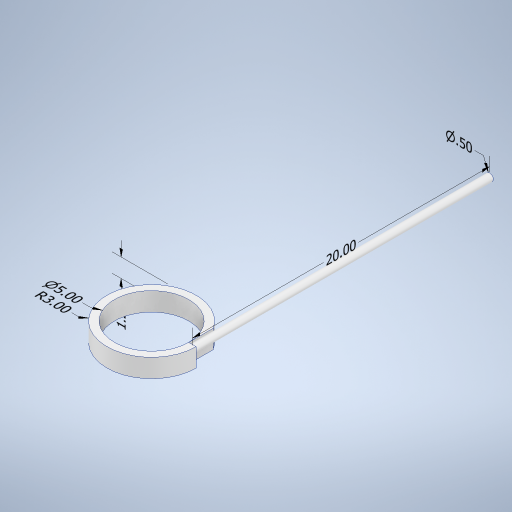
# Autodesk Inventor part: spring_180(131)
Saved by Autodesk Inventor 2024.1 (Build 281209000, 209)
## iProperties
Created: 2024-02-13
Part Number: spring_180(131)
Material: アルミニウム 6061
Document SubType Name: Modeling
Designer: hibik
Density: 2.7 g/cm^3
Appearance: アルミニウム - フラット
Author: hibik
Autodesk Inventor part; units mm, degrees
ref_plane "YZ Plane" through (0, 0, 0) normal (1, 0, 0) x (0, 1, 0)
ref_plane "XZ Plane" through (0, 0, 0) normal (0, 1, 0) x (-1, 0, 0)
ref_plane "XY Plane" through (0, 0, 0) normal (0, 0, 1) x (1, 0, 0)
sketch "スケッチ1" plane through (0, 0, 0) normal (0, 1, 0) x (-1, 0, 0)
  circle A0 centre (0, 0) radius 2.5
  circle A1 centre (0, 0) radius 3
  line L0 (-2.5, 0) -> (-3, 0)
  line L1 (-3, 0) -> (-3, -20)
  line L2 (-3, -20) -> (-2.5, -20)
  line L3 (-2.5, -20) -> (-2.5, 0)
  point P0 (-2.5, -1.6583)
  dimension "d0" = 5
  dimension "d1" = 6
  dimension "d2" = 20
  constraints: 8 end point, 2 coincident, 2 parallel, 1 centre point, 1 horizontal, 1 horizontal alignment, 1 perpendicular, 1 tangent, 1 vertical, 2 other
  measures "d1" diameter of A1
  measures "d2" distance of L0.end L1.end
extrude "押し出し1" add sketch "スケッチ1" along normal blind 1.25
sketch "スケッチ2" plane through (3, 0, -20) normal (0, 0, -1) x (-1, 0, 0)
  line L0 (0, 0) -> (0.5, 0) projected
  line L1 (0.5, 0) -> (0.5, 1.25) projected
  line L2 (0, 1.25) -> (0.5, 1.25) projected
  line L3 (0, 0) -> (0, 1.25) projected
  circle A0 centre (0.25, 1) radius 0.25
  line L4 (0, 1.25) -> (0.5, 1.25) projected
  line L5 (0.5, 0) -> (0.5, 1.25) projected
  point P0 (3, 0)
  point P1 (0, 1)
  point P2 (0.25, 1.25)
  point P3 (0.5, 1)
  constraints: 3 tangent, 1 centre point
extrude "押し出し2" cut sketch "スケッチ2" against normal blind 20 contours L3 A0 L1 L0 | L3 L2 A0 | A0 L2 L1
